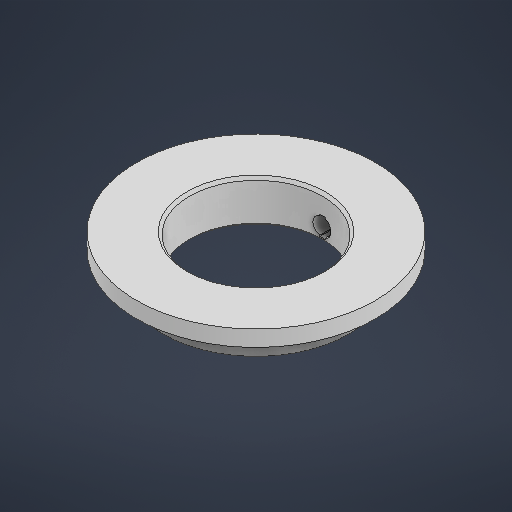
# Autodesk Inventor part: spring safety  for print
Saved by Autodesk Inventor 2025.2 (Build 292293000, 293)
## iProperties
Created: 2025-04-19
Part Number: spring safety  for print
Material: Generic
Document SubType Name: Modeling
Designer: klawy
Density: 1 g/cm^3
Appearance: Default
Author: klawy
Autodesk Inventor part; units mm, degrees
ref_plane "YZ Plane" through (0, 0, 0) normal (1, 0, 0) x (0, 1, 0)
ref_plane "XZ Plane" through (0, 0, 0) normal (0, 1, 0) x (-1, 0, 0)
sketch "Sketch1" plane through (0, 0, 0) normal (0, 0, 1) x (1, 0, 0)
  line L0 (12.54, 0) -> (22.54, 0)
  line L1 (22.54, 0) -> (22.54, 3)
  line L2 (22.54, 3) -> (12.54, 3)
  line L3 (12.54, 3) -> (12.54, 0)
  line L4 (12.54, 0) -> (17.54, 0)
  line L5 (17.54, 0) -> (17.54, -5)
  line L6 (17.54, -5) -> (12.54, -5)
  line L7 (12.54, -5) -> (12.54, 0)
  line L8 (0, -6.6) -> (0, 4.6) projected
  point P0 (0, 0)
  point P1 (17.54, 0)
  dimension "d0" = 3
  dimension "d1" = 12.54
  dimension "d2" = 10
  dimension "d3" = 5
  dimension "d4" = 5
  constraints: 16 end point, 4 parallel, 2 horizontal, 2 perpendicular, 1 point on line
  measures "d0" distance of L2.end L0.start
  measures "d1" distance from line of point (0, 0) L3
  measures "d2" distance between parallel lines of L3 L1
  measures "d3" distance of L5.end L6.end
  measures "d4" distance of L4.end L5.end
revolve "Revolution1" add sketch "Sketch1" angle 360 about axis through (0, -10, 0) along (0, 1, 0)
sketch "Sketch2" plane through (0, 0, 0) normal (0, 0, 1) x (1, 0, 0)
  line L0 (12.54, -5) -> (-12.54, -5) projected
  line L1 (12.54, 3) -> (-12.54, 3) projected
  line L2 (0, 0) -> (0, -5) construction
  point P0 (0, -2.5)
  constraints: 2 end point, 2 midpoint
hole "Hole1" at (0, -2.5, 0) direction (0, 0, -1) diameter 3.4 end through all clearance for "Hex Head Cap Screw ISO 24017" size "M3" standard "ISO"
chamfer "Chamfer1" distance 0.5 angle 45 2 edges at (-12.54, -5, 0) (-12.54, 3, 0)
ref_plane "Work Plane1" through (0, 0, -17.54) normal (0, 0, 1) x (1, 0, 0)
sketch "Sketch3" plane through (0, 0, -17.54) normal (0, 0, 1) x (1, 0, 0)
  line L0 (-0.5, -0.8752) -> (0.5, -0.8752)
  line L1 (0.5, -0.8752) -> (0.5, -4.1248)
  line L2 (0.5, -4.1248) -> (-0.5, -4.1248)
  line L3 (-0.5, -4.1248) -> (-0.5, -0.8752)
  line L4 (-0.5, -0.8752) -> (0.5, -4.1248) construction
  line L5 (0.5, -0.8752) -> (-0.5, -4.1248) construction
  line L6 (0.5, -4.1248) -> (-0.5, -4.1248)
  line L7 (-0.5, -4.1248) -> (-0.5, -4.3248)
  line L8 (-0.5, -4.3248) -> (0.5, -4.3248)
  line L9 (0.5, -4.3248) -> (0.5, -4.1248)
  line L10 (0.5, -0.8752) -> (-0.5, -0.8752)
  line L11 (-0.5, -0.8752) -> (-0.5, -0.6752)
  line L12 (-0.5, -0.6752) -> (0.5, -0.6752)
  line L13 (0.5, -0.6752) -> (0.5, -0.8752)
  point P0 (0, 0)
  point P1 (1.7, -2.5)
  point P2 (1.7, -2.5)
  point P3 (1.7, -2.5)
  point P4 (0, -2.5)
  dimension "d22" = 1
  dimension "d24" = 0.2
  dimension "d25" = 0.2
  constraints: 28 end point, 6 parallel, 3 horizontal, 3 perpendicular, 2 midpoint, 1 vertical alignment, 5 other
  measures "d22" distance of L1.end L2.end
  measures "d24" distance between parallel lines of L2 L8
  measures "d25" distance between parallel lines of L12 L0
extrude "Extrusion1" cut sketch "Sketch3" along normal blind 20 contours L11 L12 L13 L0 | L2 L9 L8 L7
body "Solid1"
